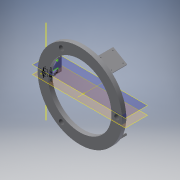
# Autodesk Inventor part: 支座
Saved by Autodesk Inventor 2017 (Build 210142000, 142)
## iProperties
Part Number: 支座
Material: 常规
Document SubType Name: Modeling
Designer: Administrator
Density: 1 g/cm^3
Appearance: 默认
Author: Administrator
Autodesk Inventor part; units mm, degrees
ref_plane "YZ Plane" through (0, 0, 0) normal (1, 0, 0) x (0, 1, 0)
ref_plane "XZ Plane" through (0, 0, 0) normal (0, 1, 0) x (-1, 0, 0)
ref_plane "XY Plane" through (0, 0, 0) normal (0, 0, 1) x (1, 0, 0)
sketch "草图1" plane through (0, 0, 0) normal (0, 1, 0) x (-1, 0, 0)
  circle A0 centre (0, 0) radius 100
  circle A1 centre (0, 0) radius 75
  dimension "d0" = 200
  dimension "d1" = 150
  constraints: 2 centre point, 2 coincident
  measures "d0" diameter of A0
  measures "d1" diameter of A1
extrude "拉伸1" add sketch "草图1" along normal blind 10
sketch "草图2" plane through (0, 10, 0) normal (0, 1, 0) x (1, 0, 0)
  line L0 (0, 0) -> (-95, 0)
  line L1 (-95, 19) -> (-95, -19)
  line L2 (-95, -19) -> (-91, -19)
  line L3 (-91, -19) -> (-91, 19)
  line L4 (-91, 19) -> (-95, 19)
  line L5 (31.0455, -91.7724) -> (63.9545, -72.7724)
  line L6 (63.9545, -72.7724) -> (61.9545, -69.3083)
  line L7 (61.9545, -69.3083) -> (29.0455, -88.3083)
  line L8 (29.0455, -88.3083) -> (31.0455, -91.7724)
  line L9 (63.9545, 72.7724) -> (31.0455, 91.7724)
  line L10 (31.0455, 91.7724) -> (29.0455, 88.3083)
  line L11 (29.0455, 88.3083) -> (61.9545, 69.3083)
  line L12 (61.9545, 69.3083) -> (63.9545, 72.7724)
  dimension "d4" = 95
  dimension "d8" = 38
  dimension "d9" = 4
  dimension "d12" = 360
  constraints: 26 end point, 2 parallel, 1 horizontal, 1 perpendicular, 1 vertical, 25 other
  measures "d4" distance of L0.start L0.end
  measures "d8" distance of L1.start L1.end
  measures "d9" distance of L2.end L1.end
extrude "拉伸2" add sketch "草图2" along normal blind 38
sketch "草图3" plane through (63.9545, 10, 72.7724) normal (0.5, 0, 0.8660254) x (0.8660254, 0, -0.5)
  line L0 (-33, 33) -> (-5, 33)
  line L1 (-5, 33) -> (-5, 5)
  line L2 (-5, 5) -> (-33, 5)
  line L3 (-33, 5) -> (-33, 33)
  line L4 (-33, 33) -> (-5, 5) construction
  line L5 (-5, 33) -> (-33, 5) construction
  circle A0 centre (-33, 33) radius 1
  circle A1 centre (-5, 33) radius 1
  circle A2 centre (-5, 5) radius 1
  circle A3 centre (-33, 5) radius 1
  point P0 (-19, -10)
  point P1 (-19, 19)
  dimension "d16" = 28
  dimension "d17" = 2
  dimension "d18" = 2
  dimension "d19" = 2
  dimension "d20" = 2
  dimension "d50" = 28
  constraints: 12 end point, 4 centre point, 4 coincident, 2 midpoint, 2 parallel, 1 horizontal, 1 perpendicular, 1 other
  measures "d16" distance of L1.end L2.end
  measures "d17" diameter of A0
  measures "d18" diameter of A1
  measures "d19" diameter of A2
  measures "d20" diameter of A3
  measures "d50" distance of L0.end L1.end
extrude "拉伸3" cut sketch "草图3" against normal through all contours L3 A0 L0 | L0 A0 L3 | A1 L1 L0 | L0 L1 A1 | A3 L2 L3 | L3 L2 A3 | A2 L2 L1 | L1 L2 A2
pattern_circular "环形阵列1" count 3 over 360 about axis through (0, 0, 0) along (0, 1, 0) of "拉伸3"
pattern_circular "环形阵列5" count 2 over 60 about axis through (0, 0, 0) along (0, 1, 0) of "拉伸2", "拉伸3", "环形阵列1"
sketch "草图10" plane through (0, 10, 0) normal (0, 1, 0) x (1, 0, 0)
  circle A0 centre (0, 0) radius 100 projected
  line L0 (0, 0) -> (0, -87.5)
  circle A1 centre (0, -87.5) radius 7
  dimension "d61" = 87.5
  dimension "d62" = 14
  constraints: 2 end point, 1 centre point, 1 coincident, 1 vertical
  measures "d61" distance of L0.start L0.end
  measures "d62" diameter of A1
extrude "拉伸8" cut sketch "草图10" against normal through all contours A1
thread "螺纹2" size "M14x2" class "6H" standard "ANSI Metric M Profile" full length
pattern_circular "环形阵列6" count 6 over 360 about axis through (0, 0, 0) along (0, 1, 0) of "拉伸8"
sketch "草图11" plane through (-95, 10, 19) normal (0, 0, 1) x (1, 0, 0)
  line L0 (4, 0) -> (4, 38) projected
  line L1 (4, 0) -> (19, 0)
  line L2 (4, 0) -> (4, 30)
  line L3 (4, 0) -> (4, 38) projected
  line L4 (4, 30) -> (19, 0)
  point P0 (95, -10)
  dimension "d78" = 15
  dimension "d79" = 30
  constraints: 6 end point, 1 horizontal, 1 point on line
  measures "d78" distance of L0.start L1.end
  measures "d79" distance of L0.start L2.end
extrude "拉伸9" add sketch "草图11" against normal blind 2
mirror "镜像1" about plane through (0, 0, 0) normal (0, 0, 1) of "拉伸9"
pattern_circular "环形阵列7" count 6 over 360 about axis through (0, 0, 0) along (0, 1, 0) of "拉伸9", "镜像1"
sketch "草图12" plane through (-91, 48, 19) normal (1, 0, 0) x (0, 0, -1)
  line L0 (0, -38) -> (7, -38)
  line L1 (36, -38) -> (2, -38) projected
  line L2 (7, -38) -> (7, -36.5)
  line L3 (7, -36.5) -> (19, -36.5)
  line L4 (19, -36.5) -> (19, -30.5)
  line L5 (19, -30.5) -> (7, -30.5)
  line L6 (7, -30.5) -> (7, -36.5)
  line L7 (0, -38) -> (8, -38)
  line L8 (8, -38) -> (8, -36)
  line L9 (8, -36) -> (18, -36)
  line L10 (18, -36) -> (18, -31)
  line L11 (18, -31) -> (8, -31)
  line L12 (8, -31) -> (8, -36)
  point P0 (19, -48)
  dimension "d85" = 7
  dimension "d86" = 1.5
  dimension "d87" = 12
  dimension "d88" = 6
  dimension "d89" = 8
  dimension "d90" = 2
  dimension "d91" = 10
  dimension "d92" = 5
  constraints: 24 end point, 4 parallel, 4 perpendicular, 2 horizontal, 2 point on line
  measures "d85" distance of L0.start L0.end
  measures "d86" distance of L0.end L2.end
  measures "d87" distance of L5.end L4.end
  measures "d88" distance of L4.end L3.end
  measures "d89" distance of L0.start L7.end
  measures "d90" distance of L7.end L8.end
  measures "d91" distance of L11.end L10.end
  measures "d92" distance of L10.end L9.end
extrude "拉伸10" cut sketch "草图12" against normal through all contours L3 L6 L5 L4 | L12 L11 L10 L9
pattern_circular "环形阵列8" count 6 over 360 about axis through (0, 0, 0) along (0, 1, 0) of "拉伸10"
thread "螺纹3" size "M2x0.4" class "6H" standard "ANSI Metric M Profile" full length
thread "螺纹4" size "M2x0.4" class "6H" standard "ANSI Metric M Profile" full length
thread "螺纹5" size "M2x0.4" class "6H" standard "ANSI Metric M Profile" full length
thread "螺纹6" size "M2x0.4" class "6H" standard "ANSI Metric M Profile" full length
thread "螺纹7" size "M2x0.4" class "6H" standard "ANSI Metric M Profile" full length
thread "螺纹8" size "M2x0.4" class "6H" standard "ANSI Metric M Profile" full length
thread "螺纹9" size "M2x0.4" class "6H" standard "ANSI Metric M Profile" full length
thread "螺纹10" size "M2x0.4" class "6H" standard "ANSI Metric M Profile" full length
thread "螺纹11" size "M2x0.4" class "6H" standard "ANSI Metric M Profile" full length
thread "螺纹12" size "M2x0.4" class "6H" standard "ANSI Metric M Profile" full length
thread "螺纹13" size "M2x0.4" class "6H" standard "ANSI Metric M Profile" full length
thread "螺纹14" size "M2x0.4" class "6H" standard "ANSI Metric M Profile" full length
thread "螺纹15" size "M2x0.4" class "6H" standard "ANSI Metric M Profile" full length
thread "螺纹16" size "M2x0.4" class "6H" standard "ANSI Metric M Profile" full length
thread "螺纹17" size "M2x0.4" class "6H" standard "ANSI Metric M Profile" full length
thread "螺纹18" size "M2x0.4" class "6H" standard "ANSI Metric M Profile" full length
thread "螺纹19" size "M2x0.4" class "6H" standard "ANSI Metric M Profile" full length
thread "螺纹20" size "M2x0.4" class "6H" standard "ANSI Metric M Profile" full length
thread "螺纹21" size "M2x0.4" class "6H" standard "ANSI Metric M Profile" full length
thread "螺纹22" size "M2x0.4" class "6H" standard "ANSI Metric M Profile" full length
thread "螺纹23" size "M2x0.4" class "6H" standard "ANSI Metric M Profile" full length
thread "螺纹24" size "M2x0.4" class "6H" standard "ANSI Metric M Profile" full length
thread "螺纹25" size "M2x0.4" class "6H" standard "ANSI Metric M Profile" full length
thread "螺纹26" size "M2x0.4" class "6H" standard "ANSI Metric M Profile" full length
